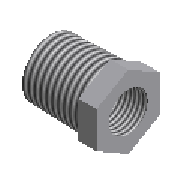
# Autodesk Inventor part: ISO 4145 Tuleja redukcyjna N4 3/8 x 1/4
Saved by Autodesk Inventor 2015 (Build 190159000, 159)
## iProperties
NAME: PIPING: ISO 4145 Reducing Bushing N4
DATA: <meta><inlinegroups number="1" deflen="1.7"></inlinegroups><connections number="2"></connections><angles><a>3.14159265358979</a></angles></meta>
Created: 2013-02-12
Part Number: ISO 4145 Tuleja redukcyjna N4 3/8 x 1/4
Material: Aluminium AW-7020
Description: ISO 4145 Elementy ze stali węglowej gwintowane zgodnie z ISO 7/1 - Tuleja redukcyjna N4
Document SubType Name: Modeling
Standard: ISO 4145
Designer: graaapsik
Standard Revision: Second edition 1986-07-15
Standards Organization: ISO
Language: pl-PL
Size Designation: 3/8 x 1/4
Categories: <MemberInstance><Categories><Category DisplayName="Rury cienko- i grubościenne" InternalName="4347fa0f-2144-441d-94cd-e3e15c92b736" Mnemonic="TUBEANDPIPE"><CategoryParameter DisplayName="GrupyWbudowane" InternalName="d60be647-bc43-4c18-a13f-9fe4115f8e64" Mnemonic="INLINEGROUPS"/><CategoryParameter DisplayName="Liczba połączeń" InternalName="04e9c83a-9e20-4a98-a7e1-e8abe87a2846" Mnemonic="NUM_CONNECTIONS"/><CategoryParameter DisplayName="Angles" InternalName="0e0e4fa4-3bd3-4656-a22e-4e07c8c476f8" Mnemonic="ANGLES"><CategoryParameter DisplayName="Angle" InternalName="9188ad83-1b16-48b4-8b0a-76ce729dafa7" Mnemonic="ANGLE"/></CategoryParameter><CategoryParameter DisplayName="NazwaElementu" InternalName="9c74ad13-48a1-45fe-b0f7-5447561f444a" Mnemonic="NAMEOFCOMPONENT"/><CategoryParameter DisplayName="KlinS" InternalName="3da84699-049a-4bc2-a65a-6696b77c242f" Mnemonic="SKEY"/><CategoryParameter DisplayName="ITEM-CODE" InternalName="99cc3b15-24d9-4d38-aac7-792cfbc57acf" Mnemonic="ITEMCODE"/><CategoryParameter DisplayName="Opis ISOGEN" InternalName="7aa3ba45-b821-4467-8584-f9e6f15f2a7d" Mnemonic="ISOGENDESC"/><Category DisplayName="Łączniki" InternalName="ed6b26c4-72b8-4f31-9b63-f85ae8f932e4" Mnemonic="FITTINGS"><CategoryParameter DisplayName="Connections" InternalName="dbd721e8-e885-4eea-9011-b5acfd9f61de" Mnemonic="FIT_CONNECTIONS"><CategoryParameter DisplayName="WielkośćZnamionowa" InternalName="3f94edc7-e459-48db-8f02-8eebf8cffccd" Mnemonic="NS"/><CategoryParameter DisplayName="KierunekPrzełączania" InternalName="d55dedc0-f14a-4283-86b4-a4eeb253c8aa" Mnemonic="FLIPDIRECTION"/><CategoryParameter DisplayName="NazwaWyświetlana" InternalName="50f521dd-e050-43f7-9895-6b30ea7ed42e" Mnemonic="DISPLAYNAME"/><CategoryParameter DisplayName="Złącze żeńskie" InternalName="b366bcb5-a500-4bad-84bb-22f956216d69" Mnemonic="FEMALE"/><CategoryParameter DisplayName="ObróbkaKońcowa" InternalName="d7f11516-3374-45ca-b1c7-4b2d63244ae2" Mnemonic="ENDTREATMENT"/><CategoryParameter DisplayName="Zamoc. na stałe" InternalName="9142902a-6a8a-446d-9eb8-4b7ce7d245ef" Mnemonic="FIXED"/><CategoryParameter DisplayName="Maks.zazębienie" InternalName="34fdf028-8797-436e-ba07-ca3dee15bd9b" Mnemonic="MAXENGAGEMENT"/><CategoryParameter DisplayName="Min.zazębienie [% maks.zazębienia]" InternalName="7ec1bde5-73f0-45b1-98d8-365a6c67f8ad" Mnemonic="MINENGAGEMENT"/><CategoryParameter DisplayName="NumerProgramuProdukcji" InternalName="d6161c62-eb59-4495-a086-874847c10866" Mnemonic="SN"/><CategoryParameter DisplayName="Maks. rozmiar rury współpracującej" InternalName="e73ef66b-c04b-45ac-9b32-f712653e25ee" Mnemonic="MXMPS"/><CategoryParameter DisplayName="Min. rozmiar rury współpracującej" InternalName="11f51b32-3e37-4310-abf7-f1318a1fd129" Mnemonic="MNMPS"/><CategoryParameter DisplayName="Wycięcie rury współpracującej" InternalName="53a63a6e-53d8-4ca9-8880-037731d1cceb" Mnemonic="CMP"/><CategoryParameter DisplayName="Obojętny rodzaj wtyku" InternalName="628bd5f1-acad-44e2-9d91-af996ab74fc2" Mnemonic="NEUTRAL"/></CategoryParameter><CategoryParameter DisplayName="Connections" InternalName="dbd721e8-e885-4eea-9011-b5acfd9f61de" Mnemonic="FIT_CONNECTIONS"><CategoryParameter DisplayName="WielkośćZnamionowa" InternalName="3f94edc7-e459-48db-8f02-8eebf8cffccd" Mnemonic="NS"/><CategoryParameter DisplayName="KierunekPrzełączania" InternalName="d55dedc0-f14a-4283-86b4-a4eeb253c8aa" Mnemonic="FLIPDIRECTION"/><CategoryParameter DisplayName="NazwaWyświetlana" InternalName="50f521dd-e050-43f7-9895-6b30ea7ed42e" Mnemonic="DISPLAYNAME"/><CategoryParameter DisplayName="Złącze żeńskie" InternalName="b366bcb5-a500-4bad-84bb-22f956216d69" Mnemonic="FEMALE"/><CategoryParameter DisplayName="ObróbkaKońcowa" InternalName="d7f11516-3374-45ca-b1c7-4b2d63244ae2" Mnemonic="ENDTREATMENT"/><CategoryParameter DisplayName="Zamoc. na stałe" InternalName="9142902a-6a8a-446d-9eb8-4b7ce7d245ef" Mnemonic="FIXED"/><CategoryParameter DisplayName="Maks.zazębienie" InternalName="34fdf028-8797-436e-ba07-ca3dee15bd9b" Mnemonic="MAXENGAGEMENT"/><CategoryParameter DisplayName="Min.zazębienie [% maks.zazębienia]" InternalName="7ec1bde5-73f0-45b1-98d8-365a6c67f8ad" Mnemonic="MINENGAGEMENT"/><CategoryParameter DisplayName="NumerProgramuProdukcji" InternalName="d6161c62-eb59-4495-a086-874847c10866" Mnemonic="SN"/><CategoryParameter DisplayName="Maks. rozmiar rury współpracującej" InternalName="e73ef66b-c04b-45ac-9b32-f712653e25ee" Mnemonic="MXMPS"/><CategoryParameter DisplayName="Min. rozmiar rury współpracującej" InternalName="11f51b32-3e37-4310-abf7-f1318a1fd129" Mnemonic="MNMPS"/><CategoryParameter DisplayName="Wycięcie rury współpracującej" InternalName="53a63a6e-53d8-4ca9-8880-037731d1cceb" Mnemonic="CMP"/><CategoryParameter DisplayName="Obojętny rodzaj wtyku" InternalName="628bd5f1-acad-44e2-9d91-af996ab74fc2" Mnemonic="NEUTRAL"/></CategoryParameter><Category DisplayName="Tuleje" InternalName="4643a10c-02fd-4de0-9209-8ad7029fa705" Mnemonic="Bushing"/></Category></Category><Category DisplayName="TypDanych" InternalName="23b78d0f-2648-40c6-8793-ca6db495c9e8" Mnemonic="DATATYPE"><CategoryParameter DisplayName="NazwaWyświetlana" InternalName="05415f3d-3907-474b-a020-eb9d644f4cf3" Mnemonic="DISPLAYNAME"/><CategoryParameter DisplayName="NazwaWewnętrzna" InternalName="cf1d0246-76d9-4b4a-8305-fa0409afb5c1" Mnemonic="INTERNALNAME"/><CategoryParameter DisplayName="Nazwa folderu" InternalName="3f06958e-8713-4116-9be7-ed6184ecc97b" Mnemonic="FOLDERNAME"/><CategoryParameter DisplayName="Wersja rodziny" InternalName="914462f6-6e19-4b14-ba84-155b9680b1d0" Mnemonic="FAMILYREVISION"/><CategoryParameter DisplayName="FormatKlipu" InternalName="bc51e27b-3422-4e78-93ef-cec197ddf230" Mnemonic="CLIPFORMAT"/><CategoryParameter DisplayName="CzyMetryczne" InternalName="e2385c5b-1ea4-4823-96a8-8de651266ec3" Mnemonic="ISMETRIC"/><CategoryParameter DisplayName="Opis" InternalName="13903e3d-64b1-4950-80da-f627842ea37f" Mnemonic="DESCRIPTION"/><CategoryParameter DisplayName="OrgStd" InternalName="8f5914e1-4693-403f-8ab5-d37768198c9d" Mnemonic="STDSORG"/><CategoryParameter DisplayName="Standardowe" InternalName="0c0a119c-1e12-4c84-803f-101930972f5e" Mnemonic="STANDARD"/><CategoryParameter DisplayName="Producent" InternalName="cd6c7a72-a28a-4e50-99a9-2c7f4e13e5ad" Mnemonic="MANUFACTURER"/><CategoryParameter DisplayName="Zmiana elementu" InternalName="a65d44b9-392f-4f4f-857b-e4b3d54996fe" Mnemonic="MEMBERREVISION"/><CategoryParameter DisplayName="Poprawka standardowa" InternalName="91d5a463-65c2-4fde-b823-3b7fea5e8e17" Mnemonic="STANDARDREVISION"/><CategoryParameter DisplayName="Wskazówki do poprawek" InternalName="45a75005-10b1-4dfc-8d6d-dfe629f0b93c" Mnemonic="REVISIONGUID"/><CategoryParameter DisplayName="Oznaczenie" InternalName="2675968c-4ce5-49e0-a4f5-552d29089031" Mnemonic="DESIGNATION"/><CategoryParameter DisplayName="Nazwa pliku" InternalName="8b46a4cc-9585-4fed-90c3-899f57e09a73" Mnemonic="FILENAME"/><CategoryParameter DisplayName="Wiersz domyślny" InternalName="2af9ec52-faaa-4026-b378-f9fa4afca842" Mnemonic="DEFAULTROW"/><Category DisplayName="Część" InternalName="c0e0b642-3bcb-4cc8-9e80-f96d35c4afa4" Mnemonic="PART"><CategoryParameter DisplayName="Materiał" InternalName="818a152a-d3c3-49ca-80ee-df7d91421b8e" Mnemonic="MATERIAL"/><CategoryParameter DisplayName="Klucz - materiał" InternalName="5c9a8adb-dd2b-4535-b97f-0a94a95fe41f" Mnemonic="MATERIALKEY"/><CategoryParameter DisplayName="Numer części" InternalName="016b6077-bfbe-49bd-92c9-d8d59c39c941" Mnemonic="PARTNUMBER"/><CategoryParameter DisplayName="Numer katalogowy" InternalName="4dba7c1c-e26c-444e-836c-b08b433409a8" Mnemonic="STOCKNUMBER"/></Category></Category><Category DisplayName="MapaPowinowactwa" InternalName="dfeab48a-acc2-4514-a11c-1b8dc28c3d5f" Mnemonic="LEGACYMAP"><CategoryParameter DisplayName="IDkatalogu" InternalName="0da51c36-8fd3-4028-86cc-0c9c9e96136a" Mnemonic="CATALOGID"/><CategoryParameter DisplayName="IDrodziny" InternalName="1c0b589c-8bbe-4e1e-80cf-07c0de42ac2a" Mnemonic="FAMILYID"/><CategoryParameter DisplayName="IDczłonka" InternalName="a368ea03-db8a-4d6e-962b-2aa46306b8f5" Mnemonic="MEMBERID"/></Category></Categories><FamilyTemplate Id="ISO 4145 Reducing Bushing N4"><FamilyTemplateParameters><FamilyTemplateParameter ObjectType="kUserParameterObject" ValueType="xs:double" Id="1" ObjectReferenceKey="MD"/><FamilyTemplateParameter ObjectType="kUserParameterObject" ValueType="xs:double" Id="2" ObjectReferenceKey="L"/><FamilyTemplateParameter ObjectType="kUserParameterObject" ValueType="xs:double" Id="3" ObjectReferenceKey="S"/><FamilyTemplateParameter ObjectType="kUserParameterObject" ValueType="xs:double" Id="4" ObjectReferenceKey="m1"/><FamilyTemplateParameter ObjectType="kUserParameterObject" ValueType="xs:double" Id="5" ObjectReferenceKey="D3"/><FamilyTemplateParameter ObjectType="kUserParameterObject" ValueType="xs:double" Id="6" ObjectReferenceKey="MjD"/><FamilyTemplateParameter ObjectType="kUserParameterObject" ValueType="xs:double" Id="7" ObjectReferenceKey="a"/><FamilyTemplateParameter ObjectType="kUserParameterObject" ValueType="xs:double" Id="116" ObjectReferenceKey="a1"/><FamilyTemplateParameter ObjectType="kUserParameterObject" ValueType="xs:string" Id="121" ObjectReferenceKey="Size_Designation"/><FamilyTemplateParameter ObjectType="kPropertyObject" ValueType="xs:string" Id="100" ObjectReferenceKey="{32853F0F-3444-11d1-9E93-0060B03C1CA6}" SubObjectId="52"/><FamilyTemplateParameter ObjectType="kPropertyObject" ValueType="xs:string" Id="105" ObjectReferenceKey="{32853F0F-3444-11d1-9E93-0060B03C1CA6}" SubObjectId="5"/><FamilyTemplateParameter ObjectType="kPartComponentDefinitionObject" ValueType="xs:string" Id="110" SubObjectId="Material"/><FamilyTemplateParameter ObjectType="kThreadFeatureObject" ValueType="xs:structure" Id="300" ObjectReferenceKey="100200001000000034090000000000008000000000000000" SubObjectId="ThreadInfo"><FamilyTemplateParameter ObjectType="" ValueType="xs:string" Id="301" SubObjectId="ThreadType"/><FamilyTemplateParameter ObjectType="" ValueType="xs:string" Id="302" SubObjectId="NominalDiameter"/></FamilyTemplateParameter><FamilyTemplateParameter ObjectType="kThreadFeatureObject" ValueType="xs:structure" Id="303" ObjectReferenceKey="1002000010000000040A0000000000008000000000000000" SubObjectId="ThreadInfo"><FamilyTemplateParameter ObjectType="" ValueType="xs:string" Id="304" SubObjectId="ThreadType"/><FamilyTemplateParameter ObjectType="" ValueType="xs:string" Id="305" SubObjectId="NominalDiameter"/></FamilyTemplateParameter></FamilyTemplateParameters></FamilyTemplate><CategoryParameterMap><ParamToTemplateMap><ParamToTemplate CategoryParameter="//CategoryParameter[@InternalName='d60be647-bc43-4c18-a13f-9fe4115f8e64']" ConstantValue="1"/><ParamToTemplate CategoryParameter="//CategoryParameter[@InternalName='04e9c83a-9e20-4a98-a7e1-e8abe87a2846']" ConstantValue="2"/><ParamToTemplate CategoryParameter="//CategoryParameter[@InternalName='0e0e4fa4-3bd3-4656-a22e-4e07c8c476f8']" ConstantValue=""/><ParamToTemplate CategoryParameter="//CategoryParameter[@InternalName='0e0e4fa4-3bd3-4656-a22e-4e07c8c476f8'][1]/CategoryParameter[@InternalName='9188ad83-1b16-48b4-8b0a-76ce729dafa7']" ConstantValue="3.14159265358979"/><ParamToTemplate CategoryParameter="//CategoryParameter[@InternalName='9c74ad13-48a1-45fe-b0f7-5447561f444a']" ConstantValue="COUPLING"/><ParamToTemplate CategoryParameter="//CategoryParameter[@InternalName='3da84699-049a-4bc2-a65a-6696b77c242f']" ConstantValue="COSC"/><ParamToTemplate CategoryParameter="//CategoryParameter[@InternalName='dbd721e8-e885-4eea-9011-b5acfd9f61de'][1]/CategoryParameter[@InternalName='d55dedc0-f14a-4283-86b4-a4eeb253c8aa']" ConstantValue="false"/><ParamToTemplate CategoryParameter="//CategoryParameter[@InternalName='dbd721e8-e885-4eea-9011-b5acfd9f61de'][1]/CategoryParameter[@InternalName='50f521dd-e050-43f7-9895-6b30ea7ed42e']" ConstantValue="Connection1"/><ParamToTemplate CategoryParameter="//CategoryParameter[@InternalName='dbd721e8-e885-4eea-9011-b5acfd9f61de'][1]/CategoryParameter[@InternalName='b366bcb5-a500-4bad-84bb-22f956216d69']" ConstantValue="false"/><ParamToTemplate CategoryParameter="//CategoryParameter[@InternalName='dbd721e8-e885-4eea-9011-b5acfd9f61de'][1]/CategoryParameter[@InternalName='d7f11516-3374-45ca-b1c7-4b2d63244ae2']" ConstantValue="Threaded"/><ParamToTemplate CategoryParameter="//CategoryParameter[@InternalName='dbd721e8-e885-4eea-9011-b5acfd9f61de'][1]/CategoryParameter[@InternalName='9142902a-6a8a-446d-9eb8-4b7ce7d245ef']" ConstantValue="false"/><ParamToTemplate CategoryParameter="//CategoryParameter[@InternalName='dbd721e8-e885-4eea-9011-b5acfd9f61de'][1]/CategoryParameter[@InternalName='34fdf028-8797-436e-ba07-ca3dee15bd9b']" ConstantValue="0"/><ParamToTemplate CategoryParameter="//CategoryParameter[@InternalName='dbd721e8-e885-4eea-9011-b5acfd9f61de'][1]/CategoryParameter[@InternalName='7ec1bde5-73f0-45b1-98d8-365a6c67f8ad']" ConstantValue="20"/><ParamToTemplate CategoryParameter="//CategoryParameter[@InternalName='dbd721e8-e885-4eea-9011-b5acfd9f61de'][2]/CategoryParameter[@InternalName='d55dedc0-f14a-4283-86b4-a4eeb253c8aa']" ConstantValue="true"/><ParamToTemplate CategoryParameter="//CategoryParameter[@InternalName='dbd721e8-e885-4eea-9011-b5acfd9f61de'][2]/CategoryParameter[@InternalName='50f521dd-e050-43f7-9895-6b30ea7ed42e']" ConstantValue="Connection2"/><ParamToTemplate CategoryParameter="//CategoryParameter[@InternalName='dbd721e8-e885-4eea-9011-b5acfd9f61de'][2]/CategoryParameter[@InternalName='b366bcb5-a500-4bad-84bb-22f956216d69']" ConstantValue="true"/><ParamToTemplate CategoryParameter="//CategoryParameter[@InternalName='dbd721e8-e885-4eea-9011-b5acfd9f61de'][2]/CategoryParameter[@InternalName='d7f11516-3374-45ca-b1c7-4b2d63244ae2']" ConstantValue="Threaded"/><ParamToTemplate CategoryParameter="//CategoryParameter[@InternalName='dbd721e8-e885-4eea-9011-b5acfd9f61de'][2]/CategoryParameter[@InternalName='9142902a-6a8a-446d-9eb8-4b7ce7d245ef']" ConstantValue="false"/><ParamToTemplate CategoryParameter="//CategoryParameter[@InternalName='dbd721e8-e885-4eea-9011-b5acfd9f61de'][2]/CategoryParameter[@InternalName='34fdf028-8797-436e-ba07-ca3dee15bd9b']" ConstantValue="0"/><ParamToTemplate CategoryParameter="//CategoryParameter[@InternalName='dbd721e8-e885-4eea-9011-b5acfd9f61de'][2]/CategoryParameter[@InternalName='7ec1bde5-73f0-45b1-98d8-365a6c67f8ad']" ConstantValue="20"/><ParamToTemplate CategoryParameter="//CategoryParameter[@InternalName='05415f3d-3907-474b-a020-eb9d644f4cf3']" ConstantValue="ISO 4145 Reducing Bushing N4"/><ParamToTemplate CategoryParameter="//CategoryParameter[@InternalName='cf1d0246-76d9-4b4a-8305-fa0409afb5c1']" ConstantValue="dd9415cf-d0a5-4cb0-ab78-dc0e0cb604b3"/><ParamToTemplate CategoryParameter="//CategoryParameter[@InternalName='3f06958e-8713-4116-9be7-ed6184ecc97b']" ConstantValue="ISO 4145 N4"/><ParamToTemplate CategoryParameter="//CategoryParameter[@InternalName='914462f6-6e19-4b14-ba84-155b9680b1d0']" ConstantValue="10"/><ParamToTemplate CategoryParameter="//CategoryParameter[@InternalName='13903e3d-64b1-4950-80da-f627842ea37f']" ConstantValue="ISO 4145 Non-alloy steel fittings threaded to ISO 7/1 - Reducing Bushing N4"/><ParamToTemplate CategoryParameter="//CategoryParameter[@InternalName='8f5914e1-4693-403f-8ab5-d37768198c9d']" ConstantValue="ISO"/><ParamToTemplate CategoryParameter="//CategoryParameter[@InternalName='0c0a119c-1e12-4c84-803f-101930972f5e']" ConstantValue="ISO 4145"/><ParamToTemplate CategoryParameter="//CategoryParameter[@InternalName='cd6c7a72-a28a-4e50-99a9-2c7f4e13e5ad']" TemplateParameter="104"/><ParamToTemplate CategoryParameter="//CategoryParameter[@InternalName='91d5a463-65c2-4fde-b823-3b7fea5e8e17']" ConstantValue="Second edition 1986-07-15"/><ParamToTemplate CategoryParameter="//CategoryParameter[@InternalName='bc51e27b-3422-4e78-93ef-cec197ddf230']" ConstantValue="CF_INVENTOR.STDPARTS"/><ParamToTemplate CategoryParameter="//CategoryParameter[@InternalName='e2385c5b-1ea4-4823-96a8-8de651266ec3']" ConstantValue="true"/><ParamToTemplate CategoryParameter="//CategoryParameter[@InternalName='45a75005-10b1-4dfc-8d6d-dfe629f0b93c']" ConstantValue="4bf51efd-3111-4f1f-a42b-a25f141ff56e"/><ParamToTemplate CategoryParameter="//CategoryParameter[@InternalName='2af9ec52-faaa-4026-b378-f9fa4afca842']" ConstantValue="1"/><ParamToTemplate CategoryParameter="//CategoryParameter[@InternalName='0da51c36-8fd3-4028-86cc-0c9c9e96136a']" ConstantValue="1B06E4C7-776A-41B3-A0ED-A3EE7199E845"/><ParamToTemplate CategoryParameter="//CategoryParameter[@InternalName='1c0b589c-8bbe-4e1e-80cf-07c0de42ac2a']" ConstantValue="dd9415cf-d0a5-4cb0-ab78-dc0e0cb604b3"/><ParamToTemplate CategoryParameter="//CategoryParameter[@InternalName='99cc3b15-24d9-4d38-aac7-792cfbc57acf']" ConstantValue=""/><ParamToTemplate CategoryParameter="//CategoryParameter[@InternalName='7aa3ba45-b821-4467-8584-f9e6f15f2a7d']" ConstantValue=""/><ParamToTemplate CategoryParameter="//CategoryParameter[@InternalName='dbd721e8-e885-4eea-9011-b5acfd9f61de'][1]/CategoryParameter[@InternalName='3f94edc7-e459-48db-8f02-8eebf8cffccd']" ConstantValue="3/8"/><ParamToTemplate CategoryParameter="//CategoryParameter[@InternalName='dbd721e8-e885-4eea-9011-b5acfd9f61de'][2]/CategoryParameter[@InternalName='3f94edc7-e459-48db-8f02-8eebf8cffccd']" ConstantValue="1/4"/><ParamToTemplate CategoryParameter="//CategoryParameter[@InternalName='8b46a4cc-9585-4fed-90c3-899f57e09a73']" ConstantValue="ISO 4145 Tuleja redukcyjna N4 3/8 x 1/4"/><ParamToTemplate CategoryParameter="//CategoryParameter[@InternalName='a65d44b9-392f-4f4f-857b-e4b3d54996fe']" ConstantValue="4f2d4fe3-0389-480c-a1cf-bdd3e3a7091f"/><ParamToTemplate CategoryParameter="//CategoryParameter[@InternalName='a368ea03-db8a-4d6e-962b-2aa46306b8f5']" ConstantValue="93DCCD4D-14C4-4AC0-8CCA-517FC8E2733D"/><ParamToTemplate CategoryParameter="//CategoryParameter[@InternalName='2675968c-4ce5-49e0-a4f5-552d29089031']" TemplateParameter="100"/><ParamToTemplate CategoryParameter="//CategoryParameter[@InternalName='818a152a-d3c3-49ca-80ee-df7d91421b8e']" TemplateParameter="110"/><ParamToTemplate CategoryParameter="//CategoryParameter[@InternalName='016b6077-bfbe-49bd-92c9-d8d59c39c941']" TemplateParameter="105"/></ParamToTemplateMap></CategoryParameterMap></MemberInstance>
Density: 2.78 g/cm^3
Appearance: Aluminium AW-7020
Mass: 5.96467 g
Surface Area: 18.6969 cm^2
Volume: 2.14557 cm^3
IsCustomPart: 0
Author: graaapsik
Autodesk Inventor part; units mm, degrees
ref_plane "YZ Plane" through (0, 0, 0) normal (1, 0, 0) x (0, 1, 0)
ref_plane "XZ Plane" through (0, 0, 0) normal (0, 1, 0) x (-1, 0, 0)
ref_plane "XY Plane" through (0, 0, 0) normal (0, 0, 1) x (1, 0, 0)
sketch "Sketch1" plane through (0, 0, 0) normal (0, 1, 0) x (-1, 0, 0)
  line L0 (0, 0) -> (-17.5, 0)
  line L1 (-17.5, 0) -> (-17.5, 5.7225) construction
  line L2 (-17.5, 8.5) -> (-12.5, 8.5)
  line L3 (-12.5, 8.5) -> (-12.5, 8.5)
  line L4 (-17.5, 8.5) -> (-17.5, 5.7225)
  line L5 (-12.5, 8.5) -> (-12.5, 8.5232)
  line L6 (-12.5, 8.5232) -> (0, 8.1326)
  line L7 (0, 8.1326) -> (0, 6.2)
  line L8 (-5.8333, 5.3579) -> (-17.5, 5.7225)
  line L9 (0, 6.2) -> (0, 0) construction
  line L10 (0, 6.2) -> (-5.8333, 6.2)
  line L11 (-5.8333, 6.2) -> (-5.8333, 5.3579)
  line L12 (-6.35, 8.331) -> (-6.35, 0) construction
  dimension "d0" = 11.445
  dimension "d1" = 17
  dimension "d4" = 17.5
  dimension "d5" = 5
  dimension "d7" = 1.79
  dimension "d9" = 12.4
  dimension "d10" = 5.8333
  dimension "d38" = 6.35
  dimension "d39" = 16.662
  constraints: 26 end point, 5 parallel, 3 perpendicular, 3 point on line, 2 horizontal, 2 vertical
  measures "d0" diameter of L1.end L0
  measures "d1" diameter of L2 L0
  measures "d4" distance of L0.start L0.end
  measures "d5" distance of L2.start L2.end
  measures "d7" angle of L0 L8
  measures "d9" diameter of L10 L0
  measures "d10" distance of L7.end L10.end
  measures "d38" distance between parallel lines of L9 L12
  measures "d39" diameter of L12.start L0
revolve "Revolve1" add sketch "Sketch1" angle 360 about axis through (0, 0, 0) along (1, 0, 0)
sketch "Sketch2" plane through (17.5, 0, 0) normal (1, 0, 0) x (0, 0, -1)
  circle A0 centre (0, 0) radius 8.5 projected
  line L0 (-8.5, 4.9075) -> (0, 9.815)
  line L1 (0, 9.815) -> (8.5, 4.9075)
  line L2 (8.5, 4.9075) -> (8.5, -4.9075)
  line L3 (8.5, -4.9075) -> (0, -9.815)
  line L4 (0, -9.815) -> (-8.5, -4.9075)
  line L5 (-8.5, -4.9075) -> (-8.5, 4.9075)
  point P0 (-8.5, 0)
  constraints: 12 end point, 1 coincident, 1 horizontal alignment, 1 midpoint, 1 vertical, 12 other
extrude "Extrude1" add sketch "Sketch2" against normal blind 5 contours L2 L3 A0 | A0 L1 L2 | A0 L0 L1 | L3 L4 A0 | A0 L5 L0 | L4 L5 A0
thread "Gwint1" size "R 3/8" standard "ISO Taper" full length
thread "Gwint2" size "Rc 1/4" standard "ISO Taper Internal" full length
equation "\"d0\" = MD"
equation "\"d1\" = S"
equation "\"d4\" = L"
equation "\"d5\" = m1"
equation "\"d9\" = D3"
equation "\"d10\" = 0.333333 * L"
equation "\"d38\" = a"
equation "\"d39\" = MjD"
equation "\"d2\" = m1"
equation "\"MD\" = 11.445"
equation "\"m1\" = 5"
equation "\"S\" = 17"
equation "\"L\" = 17.5"
equation "\"D3\" = 12.4"
equation "\"a\" = 6.35"
equation "\"MjD\" = 16.662"
equation "\"a1\" = 3.7"
equation "\"Size_Designation\" = 1.2345"
body "Solid1"
